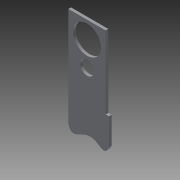
# Autodesk Inventor part: Tira
Saved by Autodesk Inventor 2015 (Build 190159000, 159)
## iProperties
Created: 2015-11-06
Part Number: Tira
Material: Generic
Document SubType Name: Modeling
Designer: EriveltonDell
Density: 1 g/cm^3
Appearance: Default
Author: EriveltonDell
Autodesk Inventor part; units mm, degrees
ref_plane "YZ Plane" through (0, 0, 0) normal (1, 0, 0) x (0, 1, 0)
ref_plane "XZ Plane" through (0, 0, 0) normal (0, 1, 0) x (-1, 0, 0)
ref_plane "XY Plane" through (0, 0, 0) normal (0, 0, 1) x (1, 0, 0)
sketch "Sketch1" plane through (0, 0, 0) normal (0, 1, 0) x (-1, 0, 0)
  circle A0 centre (0, 0) radius 5.25
  line L0 (0, 0) -> (0, 18.25)
  circle A1 centre (0, 18.25) radius 10.5
  line L1 (0, 18.25) -> (14, 18.25)
  line L2 (14, 18.25) -> (14, 31.25)
  line L3 (14, 31.25) -> (-14, 31.25)
  line L4 (-14, 31.25) -> (-14, -23.5)
  line L5 (-14, -23.5) -> (-16.5, -23.5)
  line L6 (-16.5, -23.5) -> (-16.5, -43.75)
  line L7 (14, 18.25) -> (14, -43.75)
  spline S0 degree 4 poles (14, -43.75) (9.1992, -60.1626) (-5.1458, -22.1831) (-9.6244, -59.5944) (-16.5, -43.75) knots 0 0 0 0 0 1 1 1 1 1
  point P0 (7, -47)
  point P1 (-3, -43.75)
  point P2 (-10.5, -47)
  dimension "d0" = 10.5
  dimension "d2" = 18.25
  dimension "d3" = 21
  dimension "d4" = 14
  dimension "d5" = 13
  dimension "d6" = 28
  dimension "d7" = 54.75
  dimension "d8" = 2.5
  dimension "d9" = 20.25
  dimension "d10" = 62
  constraints: 16 end point, 4 perpendicular, 3 vertical, 2 centre point, 2 coincident, 1 horizontal, 5 other
  measures "d0" diameter of A0
  measures "d2" distance of L0.start L0.end
  measures "d3" diameter of A1
  measures "d4" distance of L1.start L1.end
  measures "d5" distance of L1.end L2.end
  measures "d6" distance of L2.end L3.end
  measures "d7" distance of L3.end L4.end
  measures "d8" distance of L4.end L5.end
  measures "d9" distance of L5.end L6.end
  measures "d10" distance of L1.end L7.end
extrude "Extrusion1" add sketch "Sketch1" along normal blind 2
body "Solid1"
